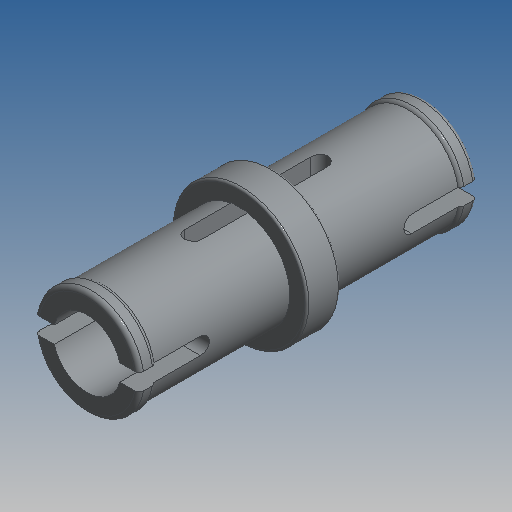
# Autodesk Inventor part: 3673-LtBluishGray
Saved by Autodesk Inventor 2022.2 (Build 262287000, 287)
## iProperties
Created: 2014-06-03
Part Number: 3673-LtBluishGray
Material: ABS Plastic
Document SubType Name: Modeling
Designer: D. Kohfeld
Appearance: LtBluishGray
Density: 1.06 g/cm^3
Mass: 0.174689 g
Surface Area: 4.61888 cm^2
Volume: 0.164801 cm^3
Author: D. Kohfeld
Autodesk Inventor part; units mm, degrees
ref_plane "YZ Plane" through (0, 0, 0) normal (1, 0, 0) x (0, 1, 0)
ref_plane "XZ Plane" through (0, 0, 0) normal (0, 1, 0) x (-1, 0, 0)
ref_plane "XY Plane" through (0, 0, 0) normal (0, 0, 1) x (1, 0, 0)
sketch "Sketch1" plane through (0, 0, 0) normal (0, 1, 0) x (-1, 0, 0)
  line L0 (2.4, 7.2) -> (2.4, 0.8)
  line L1 (3.2, 0.8) -> (2.4, 0.8)
  line L2 (3.2, 0.8) -> (3.2, -0.8)
  line L3 (2.4, -0.8) -> (3.2, -0.8)
  line L4 (2.4, -7.2) -> (2.4, -0.8)
  line L5 (2.5, 8) -> (2.5, 7.2)
  line L6 (2.5, 8) -> (1.6, 8)
  line L7 (0, -11.2) -> (0, 11.2) projected
  line L8 (2.4, 7.2) -> (2.5, 7.2)
  line L9 (1.6, 8) -> (1.6, -8)
  line L10 (3.8, 0) -> (-1.1, 0) projected
  line L11 (1.6, -8) -> (2.5, -8)
  line L12 (2.5, -8) -> (2.5, -7.2)
  line L13 (2.5, -7.2) -> (2.4, -7.2)
  line L14 (-0.4, 3) -> (-0.4, -3)
  arc A0 (-0.4, -3) -> (0.4, -3) centre (0, -3) ccw
  line L15 (0.4, -3) -> (0.4, 3)
  arc A1 (0.4, 3) -> (-0.4, 3) centre (0, 3) ccw
  point P0 (0, 0)
  point P1 (0.4, 0)
  dimension "d1" = 4.8
  dimension "d2" = 5
  dimension "d6" = 8
  dimension "d7" = 0.8
  dimension "d8" = 6.4
  dimension "d9" = 0.8
  dimension "d10" = 0.8
  dimension "d14" = 0.8
  dimension "d19" = 8
  dimension "d32" = 3.2
  dimension "d33" = 3.4
  constraints: 26 end point, 4 point on circle, 4 tangent, 3 parallel, 3 perpendicular, 2 centre point, 2 equal length, 2 point on line, 1 horizontal, 1 midpoint, 1 vertical, 1 vertical alignment, 3 other
  measures "d1" diameter of L0 L7
  measures "d2" diameter of L5 L7
  measures "d6" distance between parallel lines of L6 L10
  measures "d7" distance from line of L5.end L6
  measures "d8" diameter of L2 L7
  measures "d10" distance between parallel lines of L3 L10
  measures "d14" diameter of A1
  measures "d19" distance between parallel lines of L11 L10
  measures "d32" diameter of L9 L7
revolve "Revolution1" add sketch "Sketch1" angle 360 about axis through (0, 0, -10) along (0, 0, 1) contours L0 L1 L2 L10 L9 L6 L5 L8 | L2 L3 L4 L13 L12 L11 L9 L10
fillet "Fillet1" radius 0.2 4 edges at (2.5, 0, -7.2) (2.5, 0, -8) (2.5, 0, 8) (2.5, 0, 7.2)
fillet "Fillet1" radius 0.1 2 edges at (3.2, 0, 0.8) (3.2, 0, -0.8)
extrude "Extrusion1" cut sketch "Sketch1" along normal mid plane 4.8 contours A0 L14 L10 L7 | L7 L10 L15 A0 | L10 L14 A1 L7 | L7 A1 L15 L10
sketch "Sketch2" plane through (0, 0, 0) normal (1, 0, 0) x (0, 1, 0)
  line L0 (-1.6, 8) -> (1.6, 8) projected
  line L1 (-1.6, -8) -> (1.6, -8) projected
  line L2 (-0.4, 8) -> (0.4, 8)
  line L3 (0.4, 8) -> (0.4, 5)
  line L4 (-0.4, 5) -> (-0.4, 8)
  line L5 (0.4, -5) -> (0.4, -8)
  line L6 (0.4, -8) -> (-0.4, -8)
  line L7 (-0.4, -8) -> (-0.4, -5)
  arc A0 (0.4, -5) -> (-0.4, -5) centre (0, -5) ccw
  arc A1 (-0.4, 5) -> (0.4, 5) centre (0, 5) ccw
  point P0 (0, 0)
  point P1 (0, -8)
  point P2 (0, -8)
  point P3 (0, 8)
  dimension "d24" = 0.8
  dimension "d31" = 3.4
  constraints: 12 end point, 4 midpoint, 4 point on circle, 4 tangent, 2 centre point, 2 horizontal, 2 parallel, 2 point on line, 1 coincident, 1 collinear, 1 equal radius, 1 perpendicular, 1 vertical alignment
  measures "d24" distance of L7.end L5.start
extrude "Extrusion2" cut sketch "Sketch2" along normal through all both and the other way through all
equation "\"d1\" = tpd"
equation "\"d2\" = tpcd"
equation "\"d6\" = lu"
equation "\"d7\" = d9"
equation "\"d8\" = tsd"
equation "\"d9\" = tsl"
equation "\"d10\" = d9"
equation "\"d14\" = tpnw"
equation "\"d19\" = lu"
equation "\"d32\" = rd"
equation "\"d33\" = tpnl"
equation "\"d27\" = pinf"
equation "\"d28\" = lf"
equation "\"d24\" = tpnw"
equation "\"d31\" = tpnl"
equation "\"tpd\" = 4.8"
equation "\"tpcd\" = 5"
equation "\"lu\" = 8"
equation "\"tsd\" = 6.4"
equation "\"tsl\" = 0.8"
equation "\"tpnw\" = 0.8"
equation "\"rd\" = 3.2"
equation "\"tpnl\" = 3.4"
equation "\"pinf\" = 0.2"
equation "\"lf\" = 0.1"
body "Solid2"
